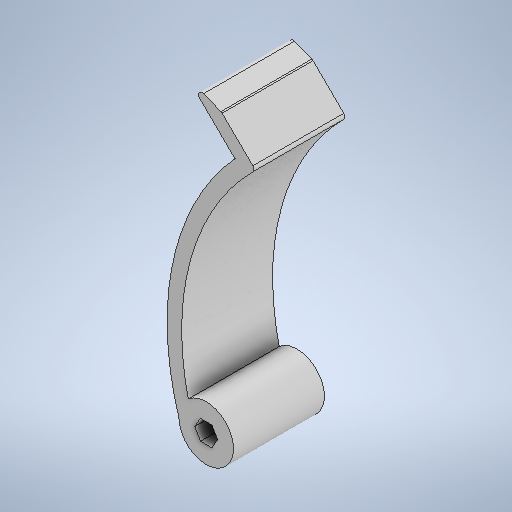
# Autodesk Inventor part: Pincer
Saved by Autodesk Inventor 2025.1 (Build 291241000, 241)
## iProperties
Created: 2024-12-07
Part Number: Pincer
Material: Generic
Document SubType Name: Modeling
Designer: ishaa
Density: 1 g/cm^3
Appearance: Default
Author: ishaa
Autodesk Inventor part; units mm, degrees
ref_plane "YZ Plane" through (0, 0, 0) normal (1, 0, 0) x (0, 1, 0)
ref_plane "XZ Plane" through (0, 0, 0) normal (0, 1, 0) x (-1, 0, 0)
ref_plane "XY Plane" through (0, 0, 0) normal (0, 0, 1) x (1, 0, 0)
sketch "Sketch1" plane through (0, 0, 0) normal (0, 0, 1) x (1, 0, 0)
  circle A0 centre (0, 0) radius 7.5
  arc A1 (7.9168, 69.2812) -> (-7.4991, -0.1156) centre (60.6498, 21.1563) ccw
  line L0 (7.9168, 69.2812) -> (-1.7941, 78.8155)
  arc A2 (12.8357, 68.6479) -> (-3.8386, 1.5889) centre (60.6498, 21.1563) ccw
  line L1 (12.8268, 70.0662) -> (4.3732, 78.366)
  line L2 (-0.7271, 80.4595) -> (4.039, 78.5829)
  arc A3 (4.3732, 78.366) -> (4.039, 78.5829) centre (3.6726, 77.6524) ccw
  arc A4 (-0.7271, 80.4595) -> (-1.7941, 78.8155) centre (-1.0935, 79.5291) ccw
  arc A5 (12.8357, 68.6479) -> (12.8268, 70.0662) centre (12.1262, 69.3526) ccw
  point P0 (-7.5, -0.0097)
  point P1 (13.5499, 69.3563)
  point P2 (-4.9334, 5.649)
  dimension "d0" = 15
  dimension "d11" = 4
  dimension "d12" = 1
  constraints: 13 point on circle, 6 centre point, 6 end point, 6 tangent, 2 equal radius, 1 coincident, 1 point on line, 1 other
  measures "d0" diameter of A0
  measures "d11" radial gap between concentric circles of A1 A2
  measures "d12" radius of A3
extrude "Extrusion1" add sketch "Sketch1" along normal blind 25
sketch "Sketch2" plane through (0, 0, 25) normal (0, 0, 1) x (1, 0, 0)
  line L0 (1.5733, 2.725) -> (3.1466, 0)
  line L1 (3.1466, 0) -> (1.5733, -2.725)
  line L2 (1.5733, -2.725) -> (-1.5733, -2.725)
  line L3 (-1.5733, -2.725) -> (-3.1466, 0)
  line L4 (-3.1466, 0) -> (-1.5733, 2.725)
  line L5 (-1.5733, 2.725) -> (1.5733, 2.725)
  point P0 (0, 0)
  point P1 (0, 0)
  dimension "d7" = 5.45
  constraints: 12 end point, 1 coincident, 13 other
  measures "d7" distance between parallel lines of L2 L5
extrude "Extrusion2" cut sketch "Sketch2" against normal blind 25
body "Solid1"
